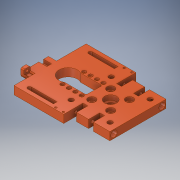
# Autodesk Inventor part: КВ33.044.901 - Щека каретки Z
Saved by Autodesk Inventor 2019 (Build 230136000, 136)
## iProperties
Created: 2019-08-08
Part Number: КВ33.044.901 - Щека каретки Z
Material: Пластик АБС
Document SubType Name: Modeling
Designer: user
Density: 1.06 g/cm^3
Appearance: Гладкий — светло-оранжевый
Mass: 66.5438 g
Surface Area: 300.742 cm^2
Volume: 62.7772 cm^3
Author: user
Autodesk Inventor part; units mm, degrees
(part 1 of 2)
ref_plane "YZ Plane" through (0, 0, 0) normal (1, 0, 0) x (0, 1, 0)
ref_plane "XZ Plane" through (0, 0, 0) normal (0, 1, 0) x (-1, 0, 0)
ref_plane "XY Plane" through (0, 0, 0) normal (0, 0, 1) x (1, 0, 0)
sketch "Эскиз4" plane through (0, 0, 0) normal (0, 1, 0) x (-1, 0, 0)
  circle A0 centre (-24.3, 25) radius 3
  circle A1 centre (24.3, 25) radius 3
  circle A2 centre (24.3, -25) radius 3
  circle A3 centre (-24.3, -25) radius 3
  line L0 (13.5, -21) -> (13.5, -35)
  line L1 (13.5, -35) -> (34, -35)
  line L2 (34, -35) -> (34, 35)
  line L3 (34, 35) -> (13.5, 35)
  line L4 (13.5, 35) -> (13.5, 21)
  line L5 (13.5, 21) -> (7.5, 21)
  line L6 (7.5, 21) -> (7.5, 35)
  line L7 (7.5, 35) -> (-7.5, 35)
  line L8 (-7.5, 35) -> (-7.5, 21)
  line L9 (-7.5, 21) -> (-13.5, 21)
  line L10 (-13.5, 21) -> (-13.5, 35)
  line L11 (-13.5, 35) -> (-34, 35)
  line L12 (-34, 35) -> (-34, -35)
  line L13 (-34, -35) -> (-13.5, -35)
  line L14 (-13.5, -35) -> (-13.5, -21)
  line L15 (-13.5, -21) -> (-7.5, -21)
  line L16 (-7.5, -21) -> (-7.5, -35)
  line L17 (-7.5, -35) -> (7.5, -35)
  line L18 (7.5, -35) -> (7.5, -21)
  line L19 (7.5, -21) -> (13.5, -21)
  circle A4 centre (0, 0) radius 7.5
  circle A5 centre (-11.749999, 11.750148) radius 4.65
  circle A6 centre (-11.750148, -11.749999) radius 4.65
  line L20 (26, 12) -> (16.393422, 12)
  line L21 (26, -12) -> (26, 12)
  line L22 (16.393281, -12) -> (26, -12)
  arc A7 (16, -9.863355) -> (16.393281, -12) centre (11.749999, -11.750148) ccw
  line L23 (16, -9.863355) -> (16, 9.86287)
  arc A8 (16.393422, 12) -> (16, 9.86287) centre (11.750148, 11.749999) ccw
  circle A9 centre (-11.749999, 11.750148) radius 2.6
  circle A10 centre (-11.750148, -11.749999) radius 2.6
  circle A11 centre (11.749999, -11.750148) radius 2.6
  circle A12 centre (11.750148, 11.749999) radius 2.6
  circle A13 centre (0, 0) radius 4.1
  circle A14 centre (11.750148, 11.749999) radius 4.65
  circle A15 centre (11.749999, -11.750148) radius 4.65
  constraints: 48 end point, 14 centre point, 4 point on circle, 2 coincident, 6 other
sketch "Эскиз4 outline for Выдавливание3" plane through (0, 0, 0) normal (0, 1, 0) x (-1, 0, 0)
  line L0 (7.5, -21) -> (13.5, -21)
  line L1 (7.5, -35) -> (7.5, -21)
  line L2 (13.5, -21) -> (13.5, -35)
  line L3 (-7.5, -35) -> (7.5, -35)
  line L4 (13.5, -35) -> (34, -35)
  line L5 (-7.5, -21) -> (-7.5, -35)
  line L6 (34, -35) -> (34, 35)
  line L7 (-13.5, -21) -> (-7.5, -21)
  line L8 (34, 35) -> (13.5, 35)
  line L9 (-13.5, -35) -> (-13.5, -21)
  line L10 (13.5, 35) -> (13.5, 21)
  line L11 (-34, -35) -> (-13.5, -35)
  line L12 (13.5, 21) -> (7.5, 21)
  line L13 (-34, 35) -> (-34, -35)
  line L14 (7.5, 21) -> (7.5, 35)
  line L15 (-13.5, 35) -> (-34, 35)
  line L16 (7.5, 35) -> (-7.5, 35)
  line L17 (-13.5, 21) -> (-13.5, 35)
  line L18 (-7.5, 35) -> (-7.5, 21)
  line L19 (-7.5, 21) -> (-13.5, 21)
  circle A0 centre (-24.3, -25) radius 3
  circle A1 centre (-11.750148, -11.749999) radius 2.6
  circle A2 centre (24.3, -25) radius 3
  circle A3 centre (11.749999, -11.750148) radius 2.6
  circle A4 centre (-11.749999, 11.750148) radius 2.6
  circle A5 centre (-24.3, 25) radius 3
  circle A6 centre (0, 0) radius 4.1
  circle A7 centre (11.750148, 11.749999) radius 2.6
  circle A8 centre (24.3, 25) radius 3
extrude "Выдавливание3" add sketch "Эскиз4 outline for Выдавливание3" along normal blind 10
sketch "Эскиз5" plane through (0, 10, 0) normal (0, 1, 0) x (1, 0, 0)
  circle A0 centre (-24.3, 25) radius 3
  circle A1 centre (24.3, 25) radius 3
  circle A2 centre (24.3, -25) radius 3
  circle A3 centre (-24.3, -25) radius 3
  line L0 (13.5, -21) -> (13.5, -35)
  line L1 (13.5, -35) -> (34, -35)
  line L2 (34, -35) -> (34, 35)
  line L3 (34, 35) -> (13.5, 35)
  line L4 (13.5, 35) -> (13.5, 21)
  line L5 (13.5, 21) -> (7.5, 21)
  line L6 (7.5, 21) -> (7.5, 35)
  line L7 (7.5, 35) -> (-7.5, 35)
  line L8 (-7.5, 35) -> (-7.5, 21)
  line L9 (-7.5, 21) -> (-13.5, 21)
  line L10 (-13.5, 21) -> (-13.5, 35)
  line L11 (-13.5, 35) -> (-34, 35)
  line L12 (-34, 35) -> (-34, -35)
  line L13 (-34, -35) -> (-13.5, -35)
  line L14 (-13.5, -35) -> (-13.5, -21)
  line L15 (-13.5, -21) -> (-7.5, -21)
  line L16 (-7.5, -21) -> (-7.5, -35)
  line L17 (-7.5, -35) -> (7.5, -35)
  line L18 (7.5, -35) -> (7.5, -21)
  line L19 (7.5, -21) -> (13.5, -21)
  circle A4 centre (0, 0) radius 7.5
  circle A5 centre (-11.749999, 11.750148) radius 4.65
  circle A6 centre (-11.750148, -11.749999) radius 4.65
  line L20 (26, 12) -> (16.393422, 12)
  line L21 (26, -12) -> (26, 12)
  line L22 (16.393281, -12) -> (26, -12)
  arc A7 (16, -9.863355) -> (16.393281, -12) centre (11.749999, -11.750148) ccw
  line L23 (16, -9.863355) -> (16, 9.86287)
  arc A8 (16.393422, 12) -> (16, 9.86287) centre (11.750148, 11.749999) ccw
  circle A9 centre (-11.749999, 11.750148) radius 2.6
  circle A10 centre (-11.750148, -11.749999) radius 2.6
  circle A11 centre (11.749999, -11.750148) radius 2.6
  circle A12 centre (11.750148, 11.749999) radius 2.6
  circle A13 centre (0, 0) radius 4.1
  circle A14 centre (11.749999, -11.750148) radius 2.6
  circle A15 centre (11.749999, -11.750148) radius 4.65
  circle A16 centre (11.750148, 11.749999) radius 4.65
  constraints: 48 end point, 16 centre point, 4 point on circle, 2 coincident, 2 concentric
sketch "Эскиз5 outline for Выдавливание4" plane through (0, 10, 0) normal (0, 1, 0) x (1, 0, 0)
  circle A0 centre (-11.749999, 11.750148) radius 4.65
  circle A1 centre (-11.749999, 11.750148) radius 2.6
  circle A2 centre (-11.750148, -11.749999) radius 4.65
  circle A3 centre (-11.750148, -11.749999) radius 2.6
  circle A4 centre (11.749999, -11.750148) radius 4.65
  circle A5 centre (11.749999, -11.750148) radius 2.6
  circle A6 centre (11.750148, 11.749999) radius 4.65
  circle A7 centre (11.750148, 11.749999) radius 2.6
extrude "Выдавливание4" cut sketch "Эскиз5 outline for Выдавливание4" against normal blind 4
sketch "Эскиз6" plane through (0, 10, 0) normal (0, 1, 0) x (1, 0, 0)
  circle A0 centre (-24.3, 25) radius 3
  circle A1 centre (24.3, 25) radius 3
  circle A2 centre (24.3, -25) radius 3
  circle A3 centre (-24.3, -25) radius 3
  line L0 (13.5, -21) -> (13.5, -35)
  line L1 (13.5, -35) -> (34, -35)
  line L2 (34, -35) -> (34, 35)
  line L3 (34, 35) -> (13.5, 35)
  line L4 (13.5, 35) -> (13.5, 21)
  line L5 (13.5, 21) -> (7.5, 21)
  line L6 (7.5, 21) -> (7.5, 35)
  line L7 (7.5, 35) -> (-7.5, 35)
  line L8 (-7.5, 35) -> (-7.5, 21)
  line L9 (-7.5, 21) -> (-13.5, 21)
  line L10 (-13.5, 21) -> (-13.5, 35)
  line L11 (-13.5, 35) -> (-34, 35)
  line L12 (-34, 35) -> (-34, -35)
  line L13 (-34, -35) -> (-13.5, -35)
  line L14 (-13.5, -35) -> (-13.5, -21)
  line L15 (-13.5, -21) -> (-7.5, -21)
  line L16 (-7.5, -21) -> (-7.5, -35)
  line L17 (-7.5, -35) -> (7.5, -35)
  line L18 (7.5, -35) -> (7.5, -21)
  line L19 (7.5, -21) -> (13.5, -21)
  circle A4 centre (0, 0) radius 7.5
  circle A5 centre (-11.749999, 11.750148) radius 4.65
  circle A6 centre (-11.750148, -11.749999) radius 4.65
  line L20 (26, 12) -> (16.393422, 12)
  line L21 (26, -12) -> (26, 12)
  line L22 (16.393281, -12) -> (26, -12)
  arc A7 (16, -9.863355) -> (16.393281, -12) centre (11.749999, -11.750148) ccw
  line L23 (16, -9.863355) -> (16, 9.86287)
  arc A8 (16.393422, 12) -> (16, 9.86287) centre (11.750148, 11.749999) ccw
  circle A9 centre (-11.749999, 11.750148) radius 2.6
  circle A10 centre (-11.750148, -11.749999) radius 2.6
  circle A11 centre (11.749999, -11.750148) radius 2.6
  circle A12 centre (11.750148, 11.749999) radius 2.6
  circle A13 centre (0, 0) radius 4.1
  constraints: 48 end point, 14 centre point, 4 point on circle
sketch "Эскиз6 outline for Выдавливание5" plane through (0, 10, 0) normal (0, 1, 0) x (1, 0, 0)
  circle A0 centre (0, 0) radius 7.5
  circle A1 centre (0, 0) radius 4.1
extrude "Выдавливание5" cut sketch "Эскиз6 outline for Выдавливание5" against normal blind 6
sketch "Эскиз7" plane through (34, 0, 35) normal (1, 0, 0) x (0, 0, -1)
  circle A0 centre (5, 5) radius 2
  circle A1 centre (5, 5) radius 4
  circle A2 centre (65, 5) radius 4
  circle A3 centre (5, 5) radius 4
  line L0 (0, 0) -> (70, 0)
  line L1 (70, 0) -> (70, 10)
  line L2 (0, 10) -> (70, 10)
  line L3 (0, 0) -> (0, 10)
  circle A4 centre (65, 5) radius 2
  circle A5 centre (65, 5) radius 4
  point P0 (35, 0)
  point P1 (35, 0)
  constraints: 8 end point, 6 centre point
sketch "Эскиз7 outline for Выдавливание6" plane through (34, 0, 35) normal (1, 0, 0) x (0, 0, -1)
  circle A0 centre (5, 5) radius 2
  circle A1 centre (65, 5) radius 2
extrude "Выдавливание6" cut sketch "Эскиз7 outline for Выдавливание6" against normal blind 269
sketch "Эскиз8" plane through (34, 0, 35) normal (1, 0, 0) x (0, 0, -1)
  circle A0 centre (5, 5) radius 2
  circle A1 centre (5, 5) radius 4
  circle A2 centre (65, 5) radius 4
  circle A3 centre (5, 5) radius 4
  line L0 (0, 0) -> (70, 0)
  line L1 (70, 0) -> (70, 10)
  line L2 (0, 10) -> (70, 10)
  line L3 (0, 0) -> (0, 10)
  circle A4 centre (65, 5) radius 2
  circle A5 centre (65, 5) radius 4
  point P0 (35, 0)
  point P1 (35, 0)
  constraints: 8 end point, 6 centre point
sketch "Эскиз8 outline for Выдавливание7" plane through (34, 0, 35) normal (1, 0, 0) x (0, 0, -1)
  circle A0 centre (5, 5) radius 4
  circle A1 centre (5, 5) radius 2
  circle A2 centre (65, 5) radius 4
  circle A3 centre (65, 5) radius 2
extrude "Выдавливание7" cut sketch "Эскиз8 outline for Выдавливание7" against normal blind 15
sketch "Эскиз9" plane through (-34, 0, -35) normal (-1, 0, 0) x (0, 0, 1)
  circle A0 centre (5, 5) radius 2
  circle A1 centre (5, 5) radius 4
  circle A2 centre (65, 5) radius 4
  circle A3 centre (5, 5) radius 4
  line L0 (0, 0) -> (70, 0)
  line L1 (70, 0) -> (70, 10)
  line L2 (0, 10) -> (70, 10)
  line L3 (0, 0) -> (0, 10)
  circle A4 centre (65, 5) radius 2
  circle A5 centre (65, 5) radius 4
  point P0 (35, 0)
  point P1 (35, 0)
  constraints: 8 end point, 6 centre point
sketch "Эскиз9 outline for Выдавливание8" plane through (-34, 0, -35) normal (-1, 0, 0) x (0, 0, 1)
  circle A0 centre (5, 5) radius 4
  circle A1 centre (5, 5) radius 2
  circle A2 centre (65, 5) radius 4
  circle A3 centre (65, 5) radius 2
extrude "Выдавливание8" cut sketch "Эскиз9 outline for Выдавливание8" against normal blind 15
sketch "Эскиз17" plane through (-34, 0, -35) normal (-1, 0, 0) x (0, 0, 1)
  line L0 (14, 10) -> (0, 10) projected
  line L1 (70, 0) -> (56, 0) projected
  line L2 (0, 10) -> (70, 10)
  line L3 (70, 10) -> (70, 0)
  line L4 (70, 0) -> (0, 0)
  line L5 (0, 0) -> (0, 10)
  point P0 (35, 0)
  constraints: 8 end point, 2 parallel, 1 horizontal, 1 perpendicular
sketch "Эскиз17 outline for Выдавливание14" plane through (-34, 0, -35) normal (-1, 0, 0) x (0, 0, 1)
  line L0 (0, 10) -> (70, 10)
  line L1 (70, 10) -> (70, 0)
  line L2 (70, 0) -> (0, 0)
  line L3 (0, 0) -> (0, 10)
extrude "Выдавливание14" add sketch "Эскиз17 outline for Выдавливание14" along normal blind 33
sketch "Эскиз18" plane through (0, 0, 0) normal (0, -1, 0) x (1, 0, 0)
  line L0 (-35.2, -12.6) -> (-35.2, -14.9)
  line L1 (-35.2, -12.6) -> (-33.8, -12.6)
  line L2 (-33.8, -14.9) -> (-33.8, -12.6)
  line L3 (-27.2, -14.9) -> (-33.8, -14.9)
  line L4 (-27.2, -12.6) -> (-27.2, -14.9)
  circle A0 centre (-53, 0) radius 9.15
  circle A1 centre (-53, 0) radius 1.5
  circle A2 centre (-17, 8) radius 1.3
  circle A3 centre (-30.5, 13.5) radius 1.3
  circle A4 centre (-22.5, 13.5) radius 1.3
  circle A5 centre (-38.5, 13.5) radius 1.3
  circle A6 centre (-46.5, 13.5) radius 1.3
  circle A7 centre (-17, -8) radius 1.3
  circle A8 centre (-30.5, -13.5) radius 1.3
  circle A9 centre (-22.5, -13.5) radius 1.3
  circle A10 centre (-38.5, -13.5) radius 1.3
  circle A11 centre (-46.5, -13.5) radius 1.3
  line L5 (-64.019804, -0.1) -> (-63.479583, -0.1)
  line L6 (-64.019804, -7) -> (-64.019804, -0.1)
  arc A12 (-64.019804, -7) -> (-63.968614, -7.75) centre (-58.5, -7) ccw
  line L7 (-61.5, -7.75) -> (-63.968614, -7.75)
  arc A13 (-59.75, -9.5) -> (-61.5, -7.75) centre (-61.5, -9.5) ccw
  line L8 (-59.75, -10) -> (-59.75, -9.5)
  line L9 (-22.193741, -10) -> (-59.75, -10)
  arc A14 (-22.193741, -10) -> (-21.505509, -9.607843) centre (-22.193741, -9.2) ccw
  arc A15 (-21.505509, -9.607843) -> (-20.892157, -8.994491) centre (-20, -10.5) ccw
  arc A16 (-20.892157, -8.994491) -> (-20.5, -8.306259) centre (-21.3, -8.306259) ccw
  line L10 (-20.5, 8.306259) -> (-20.5, -8.306259)
  arc A17 (-20.5, 8.306259) -> (-20.892157, 8.994491) centre (-21.3, 8.306259) ccw
  arc A18 (-21.505509, 9.607843) -> (-20.892157, 8.994491) centre (-20, 10.5) ccw
  arc A19 (-20.892157, 8.994491) -> (-21.505509, 9.607843) centre (-20, 10.5) ccw
  line L11 (-59.75, -11.322904) -> (-59.75, -10)
  arc A20 (-59.75, -11.322904) -> (-58.5, -11.5) centre (-58.498893, -6.992184) ccw
  line L12 (-58.5, -11.5) -> (-51, -11.5)
  line L13 (-51, -12.6) -> (-51, -11.5)
  line L14 (-49.8, -12.6) -> (-51, -12.6)
  line L15 (-49.8, -14.9) -> (-49.8, -12.6)
  line L16 (-43.2, -14.9) -> (-49.8, -14.9)
  line L17 (-43.2, -12.6) -> (-43.2, -14.9)
  line L18 (-41.8, -12.6) -> (-43.2, -12.6)
  line L19 (-41.8, -14.9) -> (-41.8, -12.6)
  line L20 (-35.2, -14.9) -> (-41.8, -14.9)
  line L21 (-35.2, -12.6) -> (-35.2, -14.9)
  line L22 (-33.8, -12.6) -> (-35.2, -12.6)
  line L23 (-33.8, -14.9) -> (-33.8, -12.6)
  line L24 (-27.2, -14.9) -> (-33.8, -14.9)
  line L25 (-27.2, -12.6) -> (-27.2, -14.9)
  line L26 (-25.8, -12.6) -> (-27.2, -12.6)
  line L27 (-25.8, -14.9) -> (-25.8, -12.6)
  line L28 (-19.2, -14.9) -> (-25.8, -14.9)
  line L29 (-19.2, -12.6) -> (-19.2, -14.9)
  line L30 (-17.980196, -12.6) -> (-19.2, -12.6)
  arc A21 (-17.980196, -12.6) -> (-17.899999, -12.519803) centre (-19, -11.5) ccw
  line L31 (-17.899999, -11.3) -> (-17.899999, -12.519803)
  line L32 (-15.6, -11.3) -> (-17.899999, -11.3)
  line L33 (-15.6, -4.7) -> (-15.6, -11.3)
  line L34 (-17.9, -4.7) -> (-15.6, -4.7)
  line L35 (-17.9, 4.7) -> (-17.9, -4.7)
  line L36 (-15.6, 4.7) -> (-17.9, 4.7)
  line L37 (-15.6, 11.3) -> (-15.6, 4.7)
  line L38 (-17.9, 11.3) -> (-15.6, 11.3)
  line L39 (-17.9, 12.519804) -> (-17.9, 11.3)
  arc A22 (-17.9, 12.519804) -> (-17.980197, 12.600001) centre (-19, 11.5) ccw
  line L40 (-19.2, 12.600001) -> (-17.980197, 12.600001)
  line L41 (-19.2, 14.9) -> (-19.2, 12.600001)
  line L42 (-25.8, 14.9) -> (-19.2, 14.9)
  line L43 (-25.8, 12.6) -> (-25.8, 14.9)
  line L44 (-27.2, 12.6) -> (-25.8, 12.6)
  line L45 (-27.2, 14.9) -> (-27.2, 12.6)
  line L46 (-33.8, 14.9) -> (-27.2, 14.9)
  line L47 (-33.8, 12.6) -> (-33.8, 14.9)
  line L48 (-35.2, 12.6) -> (-33.8, 12.6)
  line L49 (-35.2, 14.9) -> (-35.2, 12.6)
  line L50 (-41.8, 14.9) -> (-35.2, 14.9)
  line L51 (-41.8, 12.6) -> (-41.8, 14.9)
  line L52 (-43.2, 12.6) -> (-41.8, 12.6)
  line L53 (-43.2, 14.9) -> (-43.2, 12.6)
  line L54 (-49.8, 14.9) -> (-43.2, 14.9)
  line L55 (-49.8, 12.6) -> (-49.8, 14.9)
  line L56 (-51, 12.6) -> (-49.8, 12.6)
  line L57 (-51, 11.5) -> (-51, 12.6)
  line L58 (-58.5, 11.5) -> (-51, 11.5)
  arc A23 (-58.5, 11.5) -> (-59.75, 11.322904) centre (-58.498893, 6.992184) ccw
  line L59 (-59.75, 10) -> (-59.75, 11.322904)
  line L60 (-59.75, 9.5) -> (-59.75, 10)
  arc A24 (-61.5, 7.75) -> (-59.75, 9.5) centre (-61.5, 9.5) ccw
  line L61 (-63.968614, 7.75) -> (-61.5, 7.75)
  arc A25 (-63.968614, 7.75) -> (-64.019804, 7) centre (-58.5, 7) ccw
  line L62 (-64.019804, 0.1) -> (-64.019804, 7)
  line L63 (-63.479583, 0.1) -> (-64.019804, 0.1)
  arc A26 (-20.892157, -8.994491) -> (-21.505509, -9.607843) centre (-20, -10.5) ccw
  arc A27 (-21.505509, 9.607843) -> (-22.193741, 10) centre (-22.193741, 9.2) ccw
  line L64 (-59.75, 10) -> (-22.193741, 10)
  line L65 (0, 0) -> (-34, 0)
  line L66 (-34, 0) -> (-53, 0)
  line L67 (-53, -9.15) -> (-53, -10)
  line L68 (-53, 10) -> (-53, 9.15)
  dimension "d62" = 34
  dimension "d63" = 19
  constraints: 138 end point, 34 point on circle, 28 centre point, 4 point on line, 2 horizontal, 1 perpendicular
  measures "d62" distance of L65.start L65.end
  measures "d63" distance of L65.end L66.end
sketch "Эскиз18 outline for Выдавливание15" plane through (0, 0, 0) normal (0, -1, 0) x (1, 0, 0)
  arc A0 (-53, 9.15) -> (-53, -9.15) centre (-53, 0) ccw
  line L0 (-53, -9.15) -> (-53, -10)
  line L1 (-53, -10) -> (-22.193741, -10)
  arc A1 (-22.193741, -10) -> (-21.505509, -9.607843) centre (-22.193741, -9.2) ccw
  arc A2 (-21.505509, -9.607843) -> (-20.892157, -8.994491) centre (-20, -10.5) cw
  arc A3 (-20.892157, -8.994491) -> (-20.5, -8.306259) centre (-21.3, -8.306259) ccw
  line L2 (-20.5, -8.306259) -> (-20.5, 8.306259)
  arc A4 (-20.5, 8.306259) -> (-20.892157, 8.994491) centre (-21.3, 8.306259) ccw
  arc A5 (-20.892157, 8.994491) -> (-21.505509, 9.607843) centre (-20, 10.5) cw
  arc A6 (-21.505509, 9.607843) -> (-22.193741, 10) centre (-22.193741, 9.2) ccw
  line L3 (-22.193741, 10) -> (-53, 10)
  line L4 (-53, 10) -> (-53, 9.15)
  circle A7 centre (-30.5, 13.5) radius 1.3
  circle A8 centre (-22.5, 13.5) radius 1.3
  circle A9 centre (-38.5, 13.5) radius 1.3
  circle A10 centre (-46.5, 13.5) radius 1.3
  circle A11 centre (-30.5, -13.5) radius 1.3
  circle A12 centre (-22.5, -13.5) radius 1.3
  circle A13 centre (-38.5, -13.5) radius 1.3
  circle A14 centre (-46.5, -13.5) radius 1.3
extrude "Выдавливание15" cut sketch "Эскиз18 outline for Выдавливание15" against normal blind 23
sketch "Эскиз19" plane through (0, 0, 0) normal (0, -1, 0) x (1, 0, 0)
  arc A0 (-53, 9.15) -> (-53, -9.15) centre (-53, 0) ccw projected
  circle A1 centre (-53, 0) radius 11.5
  point P0 (0, 0)
  dimension "d66" = 23
  constraints: 1 centre point, 1 coincident
  measures "d66" diameter of A1
sketch "Эскиз19 outline for Выдавливание16" plane through (0, 0, 0) normal (0, -1, 0) x (1, 0, 0)
  circle A0 centre (-53, 0) radius 11.5
extrude "Выдавливание16" cut sketch "Эскиз19 outline for Выдавливание16" against normal blind 23
sketch "Эскиз20" plane through (0, 10, 0) normal (0, 1, 0) x (1, 0, 0)
  circle A0 centre (-22.5, -13.5) radius 1.3 projected
  circle A1 centre (-22.5, -13.5) radius 2.5
  circle A2 centre (-30.5, -13.5) radius 1.3 projected
  circle A3 centre (-30.5, -13.5) radius 2.5
  circle A4 centre (-38.5, -13.5) radius 1.3 projected
  circle A5 centre (-38.5, -13.5) radius 2.5
  circle A6 centre (-46.5, -13.5) radius 1.3 projected
  circle A7 centre (-46.5, -13.5) radius 2.5
  circle A8 centre (-46.5, 13.5) radius 1.3 projected
  circle A9 centre (-46.5, 13.5) radius 2.5
  circle A10 centre (-38.5, 13.5) radius 1.3 projected
  circle A11 centre (-38.5, 13.5) radius 2.5
  circle A12 centre (-30.5, 13.5) radius 1.3 projected
  circle A13 centre (-30.5, 13.5) radius 2.5
  circle A14 centre (-22.5, 13.5) radius 1.3 projected
  circle A15 centre (-22.5, 13.5) radius 2.5
  point P0 (0, 0)
  dimension "d69" = 5
  dimension "d70" = 5
  dimension "d71" = 5
  dimension "d72" = 5
  dimension "d73" = 5
  dimension "d74" = 5
  dimension "d75" = 5
  dimension "d76" = 5
  constraints: 8 centre point, 8 coincident
  measures "d69" diameter of A1
  measures "d70" diameter of A3
  measures "d71" diameter of A5
  measures "d72" diameter of A7
  measures "d73" diameter of A9
  measures "d74" diameter of A11
  measures "d75" diameter of A13
  measures "d76" diameter of A15
sketch "Эскиз20 outline for Выдавливание17" plane through (0, 10, 0) normal (0, 1, 0) x (1, 0, 0)
  circle A0 centre (-22.5, -13.5) radius 2.5
  circle A1 centre (-30.5, -13.5) radius 2.5
  circle A2 centre (-38.5, -13.5) radius 2.5
  circle A3 centre (-46.5, -13.5) radius 2.5
  circle A4 centre (-46.5, 13.5) radius 2.5
  circle A5 centre (-38.5, 13.5) radius 2.5
  circle A6 centre (-30.5, 13.5) radius 2.5
  circle A7 centre (-22.5, 13.5) radius 1.3
extrude "Выдавливание17" cut sketch "Эскиз20 outline for Выдавливание17" against normal blind 2
move faces "Перенос3" translate (0, 0, -10) faces at (-49.166667, 6.666667, -35)
move faces "Перенос4" translate (0, 0, 10) faces at (-31.333333, 6.666667, 35)
sketch "Эскиз21" plane through (0, 10, 0) normal (0, 1, 0) x (1, 0, 0)
  line L0 (-13.5, -45) -> (-67, -45)
  line L1 (-40.25, -45) -> (-40.25, -38)
  line L2 (-13.5, 45) -> (-67, 45)
  line L3 (-40.25, 45) -> (-40.25, 38)
  line L4 (-17.168403, -38) -> (-63.331597, -38) construction
  line L5 (-17.168403, -35.75) -> (-63.331597, -35.75)
  line L6 (-63.331597, -40.25) -> (-17.168403, -40.25)
  arc A0 (-17.168403, -40.25) -> (-17.168403, -35.75) centre (-17.168403, -38) ccw
  arc A1 (-63.331597, -35.75) -> (-63.331597, -40.25) centre (-63.331597, -38) ccw
  line L7 (-17.168403, 38) -> (-63.331597, 38) construction
  line L8 (-17.168403, 40.25) -> (-63.331597, 40.25)
  line L9 (-63.331597, 35.75) -> (-17.168403, 35.75)
  arc A2 (-17.168403, 35.75) -> (-17.168403, 40.25) centre (-17.168403, 38) ccw
  arc A3 (-63.331597, 40.25) -> (-63.331597, 35.75) centre (-63.331597, 38) ccw
  point P0 (0, 0)
  dimension "d85" = 7
  dimension "d86" = 7
  dimension "d87" = 90
  dimension "d88" = 4.5
  dimension "d89" = 4.5
  constraints: 20 end point, 8 point on circle, 8 tangent, 4 centre point, 4 midpoint, 2 horizontal, 2 parallel, 1 vertical
  measures "d85" distance of L1.start L1.end
  measures "d86" distance of L3.start L3.end
  measures "d87" angle of L2 L3
  measures "d88" diameter of A1
  measures "d89" diameter of A3
sketch "Эскиз21 outline for Выдавливание18" plane through (0, 10, 0) normal (0, 1, 0) x (1, 0, 0)
  arc A0 (-17.168403, -40.25) -> (-17.168403, -35.75) centre (-17.168403, -38) ccw
  line L0 (-63.331597, -40.25) -> (-17.168403, -40.25)
  arc A1 (-63.331597, -35.75) -> (-63.331597, -40.25) centre (-63.331597, -38) ccw
  line L1 (-17.168403, -35.75) -> (-63.331597, -35.75)
  arc A2 (-17.168403, 35.75) -> (-17.168403, 40.25) centre (-17.168403, 38) ccw
  line L2 (-63.331597, 35.75) -> (-17.168403, 35.75)
  arc A3 (-63.331597, 40.25) -> (-63.331597, 35.75) centre (-63.331597, 38) ccw
  line L3 (-17.168403, 40.25) -> (-63.331597, 40.25)
extrude "Выдавливание18" cut sketch "Эскиз21 outline for Выдавливание18" against normal blind 15.5
move faces "Перенос5" translate (-8.5, 0, 0) faces at (-67, 3.333333, 15)
sketch "Эскиз24" plane through (-75.5, 0, -45) normal (-1, 0, 0) x (0, 0, 1)
  line L0 (90, 0) -> (90, 10) projected
  line L1 (90, 0) -> (66, 0) projected
  line L2 (90, 0) -> (90, 5.8)
  line L3 (90, 5.8) -> (49.1, 5.8)
  line L4 (49.1, 5.8) -> (90, 5.8)
  line L5 (90, 5.8) -> (90, 10)
  line L6 (90, 10) -> (49.1, 10)
  line L7 (49.1, 10) -> (49.1, 5.8)
  line L8 (49.1, 10) -> (71.6, 10)
  line L9 (90, 10) -> (0, 10) projected
  line L10 (71.6, 10) -> (71.6, 5.8)
  point P0 (45, 0)
  dimension "d103" = 5.8
  dimension "d104" = 40.9
  dimension "d105" = 22.5
  constraints: 16 end point, 3 perpendicular, 3 point on line, 2 parallel, 1 horizontal
  measures "d103" distance of L0.start L2.end
  measures "d104" distance of L2.end L3.end
  measures "d105" distance of L6.end L8.end
sketch "Эскиз24 outline for Выдавливание20" plane through (-75.5, 0, -45) normal (-1, 0, 0) x (0, 0, 1)
  line L0 (49.1, 10) -> (49.1, 5.8)
  line L1 (71.6, 10) -> (49.1, 10)
  line L2 (71.6, 5.8) -> (71.6, 10)
  line L3 (49.1, 5.8) -> (71.6, 5.8)
extrude "Выдавливание20" add sketch "Эскиз24 outline for Выдавливание20" along normal blind 10
sketch "Эскиз25" plane through (-75.5, 0, -45) normal (-1, 0, 0) x (0, 0, 1)
  line L0 (49.1, 5.8) -> (49.1, 10)
  line L1 (49.1, 5.8) -> (43.1, 5.8)
  line L2 (43.1, 5.8) -> (43.1, 0)
  line L3 (43.1, 0) -> (49.1, 0)
  line L4 (49.1, 0) -> (49.1, 5.8)
  line L5 (43.1, 5.8) -> (37.1, 5.8)
  line L6 (37.1, 5.8) -> (37.1, 10)
  line L7 (37.1, 10) -> (43.1, 10)
  line L8 (43.1, 10) -> (43.1, 5.8)
  line L9 (41.995544, 5.8) -> (43.1, 4.63325)
  line L10 (49.1, 4.63325) -> (50.332559, 5.8)
  line L11 (71.6, 5.8) -> (49.1, 5.8)
  line L12 (49.1, 5.8) -> (50.332559, 5.8)
  point P0 (45, 0)
  dimension "d108" = 6
  dimension "d109" = 5.8
  dimension "d110" = 6
  dimension "d111" = 4.2
  constraints: 22 end point, 4 parallel, 4 point on line, 3 horizontal, 3 perpendicular
  measures "d108" distance of L3.end L2.end
  measures "d109" distance of L2.end L1.end
  measures "d110" distance of L6.end L7.end
  measures "d111" distance of L5.end L6.end
sketch "Эскиз25 outline for Выдавливание21" plane through (-75.5, 0, -45) normal (-1, 0, 0) x (0, 0, 1)
  line L0 (41.995544, 5.8) -> (43.1, 4.63325)
  line L1 (43.1, 4.63325) -> (43.1, 0)
  line L2 (43.1, 0) -> (49.1, 0)
  line L3 (49.1, 0) -> (49.1, 4.63325)
  line L4 (49.1, 4.63325) -> (50.332559, 5.8)
  line L5 (50.332559, 5.8) -> (43.1, 5.8)
  line L6 (43.1, 5.8) -> (43.1, 10)
  line L7 (43.1, 10) -> (37.1, 10)
  line L8 (37.1, 10) -> (37.1, 5.8)
  line L9 (37.1, 5.8) -> (41.995544, 5.8)
extrude "Выдавливание21" add sketch "Эскиз25 outline for Выдавливание21" along normal blind 10
sketch "Эскиз26" plane through (-85.5, 0, -45) normal (-1, 0, 0) x (0, 0, 1)
  line L0 (71.6, 5.8) -> (71.6, 10) projected
  line L1 (71.6, 7.9) -> (67.5, 7.9)
  line L2 (71.6, 5.8) -> (63.6, 5.8)
  line L3 (63.6, 5.8) -> (63.6, 15.1)
  line L4 (63.6, 15.1) -> (71.6, 15.1)
  line L5 (71.6, 15.1) -> (71.6, 5.8)
  line L6 (67.5, 7.9) -> (67.5, 11.7)
  circle A0 centre (67.5, 11.7) radius 1.5
  point P0 (45, 0)
  dimension "d114" = 4.1
  dimension "d115" = 8
  dimension "d116" = 9.3
  dimension "d117" = 3.8
  dimension "d118" = 3
  constraints: 12 end point, 2 horizontal, 2 parallel, 1 centre point, 1 coincident, 1 midpoint, 1 perpendicular, 1 vertical
  measures "d114" distance of L1.start L1.end
  measures "d115" distance of L3.end L4.end
  measures "d116" distance of L2.end L3.end
  measures "d117" distance of L1.end L6.end
  measures "d118" diameter of A0
sketch "Эскиз26 outline for Выдавливание22" plane through (-85.5, 0, -45) normal (-1, 0, 0) x (0, 0, 1)
  line L0 (63.6, 5.8) -> (71.6, 5.8)
  line L1 (63.6, 15.1) -> (63.6, 5.8)
  line L2 (71.6, 5.8) -> (71.6, 15.1)
  line L3 (71.6, 15.1) -> (63.6, 15.1)
  circle A0 centre (67.5, 11.7) radius 1.5
extrude "Выдавливание22" add sketch "Эскиз26 outline for Выдавливание22" against normal blind 4
sketch "Эскиз29" plane through (0, 10, 0) normal (0, 1, 0) x (1, 0, 0)
  line L0 (-81.5, -21) -> (-81.5, -24)
  line L1 (-81.5, -21) -> (-81.5, -20)
  line L2 (-81.5, -18.6) -> (-81.5, -26.6)
  line L3 (-75.5, -26.6) -> (-75.5, -5.332559)
  line L4 (-81.5, -20) -> (-75.5, -20)
  line L5 (-75.5, -20) -> (-75.5, -25)
  line L6 (-75.5, -25) -> (-81.5, -25)
  line L7 (-81.5, -25) -> (-81.5, -20)
  point P0 (0, 0)
  dimension "d127" = 1
  dimension "d128" = 5
  constraints: 10 end point, 2 parallel, 2 point on line, 1 horizontal, 1 perpendicular
  measures "d127" distance of L0.start L1.end
  measures "d128" distance of L4.end L5.end
sketch "Эскиз29 outline for Выдавливание25" plane through (0, 10, 0) normal (0, 1, 0) x (1, 0, 0)
  line L0 (-75.5, -20) -> (-81.5, -20)
  line L1 (-75.5, -25) -> (-75.5, -20)
  line L2 (-81.5, -25) -> (-75.5, -25)
  line L3 (-81.5, -20) -> (-81.5, -25)
extrude "Выдавливание25" cut sketch "Эскиз29 outline for Выдавливание25" against normal blind 2
chamfer "Фаска2" distance 1.25 angle 45 2 edges at (-78.5, 10, 20) (-78.5, 10, 25)
chamfer "Фаска3" distance 1.25 angle 45 2 edges at (-83.5, 15.1, 26.6) (-83.5, 15.1, 18.6)
sketch "Эскиз30" plane through (-75.5, 0, 45) normal (-1, 0, 0) x (0, 0, 1)
  circle A0 centre (-15, 5) radius 2 projected
  circle A1 centre (-15, 5) radius 4
  circle A2 centre (-75, 5) radius 2 projected
  circle A3 centre (-75, 5) radius 4
  point P0 (-45, 0)
  constraints: 2 centre point, 2 coincident
sketch "Эскиз30 outline for Выдавливание26" plane through (-75.5, 0, 45) normal (-1, 0, 0) x (0, 0, 1)
  circle A0 centre (-15, 5) radius 4
  circle A1 centre (-75, 5) radius 4
extrude "Выдавливание26" cut sketch "Эскиз30 outline for Выдавливание26" against normal blind 56.25 and the other way blind 12.125
sketch "Эскиз32" plane through (0, 0, 0) normal (0, -1, 0) x (1, 0, 0)
  line L0 (-13.5, -21) -> (-13.5, -45)
  line L1 (-13.5, -45) -> (-31.053592, -45)
  line L2 (-31.053592, -45) -> (-31.053592, -35.241695)
  line L3 (-31.053592, -35.241695) -> (-13.5, -35.241695)
  line L4 (-13.5, -35.241695) -> (-13.5, -45)
  line L5 (-13.5, 45) -> (-31.053592, 45)
  line L6 (-31.053592, 45) -> (-31.053592, 35)
  line L7 (-31.053592, 35) -> (-13.5, 35)
  line L8 (-13.5, 35) -> (-13.5, 45)
  point P0 (0, 0)
  dimension "d145" = 10
  constraints: 16 end point, 4 parallel, 2 horizontal, 2 perpendicular, 1 point on line
  measures "d145" distance of L7.end L5.start
sketch "Эскиз32 outline for Выдавливание27" plane through (0, 0, 0) normal (0, -1, 0) x (1, 0, 0)
  line L0 (-13.5, -45) -> (-31.053592, -45)
  line L1 (-31.053592, -45) -> (-31.053592, -35.241695)
  line L2 (-31.053592, -35.241695) -> (-13.5, -35.241695)
  line L3 (-13.5, -35.241695) -> (-13.5, -45)
  line L4 (-13.5, 35) -> (-13.5, 45)
  line L5 (-31.053592, 35) -> (-13.5, 35)
  line L6 (-31.053592, 45) -> (-31.053592, 35)
  line L7 (-13.5, 45) -> (-31.053592, 45)
extrude "Выдавливание27" add sketch "Эскиз32 outline for Выдавливание27" against normal blind 10
sketch "Эскиз31" plane through (0, 0, 0) normal (0, -1, 0) x (1, 0, 0)
  line L0 (-11.162974, 50.524965) -> (-11.675559, 50.524965)
  line L1 (-11.675559, 50.524965) -> (-11.767254, 49.090957)
  arc A0 (-15.958694, 49.090957) -> (-11.767254, 49.090957) centre (-13.862974, 49.224965) ccw
  line L2 (-15.958694, 49.090957) -> (-16.05039, 50.524965)
  line L3 (-16.05039, 50.524965) -> (-20.33871, 50.524965)
  arc A1 (-20.33871, 50.524965) -> (-20.409421, 50.495675) centre (-20.33871, 50.424965) ccw
  line L4 (-20.409421, 50.495675) -> (-20.733685, 50.171411)
  arc A2 (-21.087238, 50.024965) -> (-20.733685, 50.171411) centre (-21.087238, 50.524965) ccw
  line L5 (-21.087238, 50.024965) -> (-30.762974, 50.024965)
  arc A3 (-30.762974, 50.024965) -> (-30.862974, 49.924965) centre (-30.762974, 49.924965) ccw
  line L6 (-30.862974, 49.924965) -> (-30.862974, 40.774965)
  arc A4 (-30.862974, 40.774965) -> (-30.762974, 40.674965) centre (-30.762974, 40.774965) ccw
  line L7 (-30.762974, 40.674965) -> (-27.837238, 40.674965)
  arc A5 (-27.483685, 40.528518) -> (-27.837238, 40.674965) centre (-27.837238, 40.174965) ccw
  line L8 (-27.483685, 40.528518) -> (-27.159421, 40.204254)
  arc A6 (-27.159421, 40.204254) -> (-27.08871, 40.174965) centre (-27.08871, 40.274965) ccw
  line L9 (-27.08871, 40.174965) -> (-24.337238, 40.174965)
  arc A7 (-24.337238, 40.174965) -> (-24.266528, 40.204254) centre (-24.337238, 40.274965) ccw
  line L10 (-24.266528, 40.204254) -> (-23.942264, 40.528518)
  arc A8 (-23.58871, 40.674965) -> (-23.942264, 40.528518) centre (-23.58871, 40.174965) ccw
  line L11 (-23.58871, 40.674965) -> (-18.337238, 40.674965)
  arc A9 (-17.983685, 40.528518) -> (-18.337238, 40.674965) centre (-18.337238, 40.174965) ccw
  line L12 (-17.983685, 40.528518) -> (-17.659421, 40.204254)
  arc A10 (-17.659421, 40.204254) -> (-17.58871, 40.174965) centre (-17.58871, 40.274965) ccw
  line L13 (-17.58871, 40.174965) -> (-14.837238, 40.174965)
  arc A11 (-14.837238, 40.174965) -> (-14.766528, 40.204254) centre (-14.837238, 40.274965) ccw
  line L14 (-14.766528, 40.204254) -> (-14.442264, 40.528518)
  arc A12 (-14.08871, 40.674965) -> (-14.442264, 40.528518) centre (-14.08871, 40.174965) ccw
  line L15 (-14.08871, 40.674965) -> (-11.162974, 40.674965)
  arc A13 (-11.162974, 40.674965) -> (-11.062974, 40.774965) centre (-11.162974, 40.774965) ccw
  line L16 (-11.062974, 40.774965) -> (-11.062974, 50.424965)
  arc A14 (-11.062974, 50.424965) -> (-11.162974, 50.524965) centre (-11.162974, 50.424965) ccw
  circle A15 centre (-16.212974, 42.724965) radius 1.25
  circle A16 centre (-25.712974, 42.724965) radius 1.25
  line L17 (-26.886308, 44.974965) -> (-26.269641, 46.274965)
  line L18 (-26.269641, 46.274965) -> (-26.252974, 46.274965)
  line L19 (-26.252974, 46.274965) -> (-25.652974, 44.974965)
  line L20 (-25.652974, 44.974965) -> (-25.779797, 44.974965)
  line L21 (-25.779797, 44.974965) -> (-25.971985, 45.391631)
  line L22 (-25.971985, 45.391631) -> (-26.561308, 45.391631)
  line L23 (-26.561308, 45.391631) -> (-26.758964, 44.974965)
  line L24 (-26.758964, 44.974965) -> (-26.886308, 44.974965)
  spline S0 degree 3 poles (-24.066308, 45.911423) (-24.066544, 45.920293) (-24.067009, 45.937775) (-24.071116, 45.963406) (-24.077323, 45.98813) (-24.086217, 46.012023) (-24.097957, 46.034846) (-24.112247, 46.056625) (-24.128734, 46.077681) (-24.147808, 46.097424) (-24.168761, 46.115506) (-24.190896, 46.131523) (-24.214314, 46.144909) (-24.238918, 46.155882) (-24.264637, 46.16449) (-24.291523, 46.170455) (-24.319501, 46.1742) (-24.338605, 46.174707) (-24.348339, 46.174965) knots 0 0 0 0 0.0619654 0.12212191 0.1809885 0.23993322 0.29990583 0.35998885 0.42177574 0.48657583 0.5515348 0.61501754 0.67725862 0.73972996 0.8030501 0.86649513 0.93197347 1 1 1 1
  spline S1 degree 3 poles (-24.348339, 46.174965) (-24.358505, 46.174699) (-24.37847, 46.174178) (-24.407783, 46.170529) (-24.435746, 46.164235) (-24.46243, 46.155627) (-24.48788, 46.144685) (-24.511973, 46.131056) (-24.534653, 46.114794) (-24.555965, 46.096356) (-24.5756, 46.075828) (-24.592851, 46.052944) (-24.607926, 46.028123) (-24.621078, 46.00143) (-24.631758, 45.972625) (-24.63992, 45.941808) (-24.646378, 45.909114) (-24.648535, 45.886537) (-24.649641, 45.874965) knots 0 0 0 0 0.06443867 0.12654691 0.18688715 0.24587754 0.30404088 0.36219122 0.42097593 0.48066028 0.54060027 0.6006891 0.66193579 0.72444251 0.78903839 0.85631376 0.92635203 1 1 1 1
  line L25 (-24.649641, 45.874965) -> (-24.766308, 45.874965)
  spline S2 degree 3 poles (-24.766308, 45.874965) (-24.765547, 45.890443) (-24.764054, 45.92084) (-24.757061, 45.965161) (-24.747054, 46.007524) (-24.732906, 46.04759) (-24.715335, 46.085713) (-24.694264, 46.121741) (-24.669306, 46.155538) (-24.641001, 46.18679) (-24.610258, 46.215459) (-24.577087, 46.240217) (-24.54223, 46.261135) (-24.505793, 46.278622) (-24.467365, 46.291749) (-24.427294, 46.301488) (-24.385405, 46.307348) (-24.356865, 46.307978) (-24.342349, 46.308298) knots 0 0 0 0 0.06879079 0.13510329 0.19897867 0.2619043 0.32349497 0.38519538 0.44696924 0.50976478 0.57225057 0.63340518 0.69325116 0.75258316 0.81257927 0.87327508 0.93554994 1 1 1 1
  spline S3 degree 3 poles (-24.342349, 46.308298) (-24.328095, 46.307964) (-24.300085, 46.307309) (-24.259204, 46.301677) (-24.220287, 46.292858) (-24.183409, 46.280483) (-24.148864, 46.263849) (-24.116392, 46.243867) (-24.085608, 46.220757) (-24.057897, 46.193548) (-24.032451, 46.164502) (-24.010499, 46.133492) (-23.9917, 46.101464) (-23.97603, 46.068173) (-23.964495, 46.033307) (-23.955737, 45.997372) (-23.950787, 45.959998) (-23.950027, 45.934701) (-23.949641, 45.92184) knots 0 0 0 0 0.06947546 0.1365168 0.20078882 0.26382967 0.32573502 0.38729069 0.44950922 0.51296782 0.57627522 0.6375801 0.69790261 0.75717209 0.81659853 0.87665317 0.93728964 1 1 1 1
  spline S4 degree 3 poles (-23.949641, 45.92184) (-23.95027, 45.903733) (-23.951517, 45.867838) (-23.962182, 45.81509) (-23.978839, 45.763984) (-23.998895, 45.722853) (-24.019128, 45.689709) (-24.037361, 45.662421) (-24.058705, 45.633039) (-24.083471, 45.601661) (-24.111147, 45.568043) (-24.141984, 45.532204) (-24.176201, 45.494514) (-24.200217, 45.468772) (-24.212662, 45.455434) knots 0 0 0 0 0.0987022 0.19567231 0.29242243 0.39134254 0.44446244 0.50422878 0.57035234 0.64254575 0.72228751 0.80792112 0.90046954 1 1 1 1
  line L26 (-24.212662, 45.455434) -> (-24.537922, 45.108298)
  line L27 (-24.537922, 45.108298) -> (-23.932974, 45.108298)
  line L28 (-23.932974, 45.108298) -> (-23.932974, 44.974965)
  line L29 (-23.932974, 44.974965) -> (-24.816308, 44.974965)
  line L30 (-24.816308, 44.974965) -> (-24.312141, 45.512986)
  spline S5 degree 3 poles (-24.312141, 45.512986) (-24.299866, 45.525799) (-24.276288, 45.550412) (-24.242941, 45.586345) (-24.212989, 45.61968) (-24.18624, 45.650355) (-24.163273, 45.678818) (-24.142892, 45.704148) (-24.126562, 45.727457) (-24.108839, 45.754475) (-24.091674, 45.787462) (-24.076923, 45.827775) (-24.067929, 45.869273) (-24.06685, 45.897317) (-24.066308, 45.911423) knots 0 0 0 0 0.11080264 0.2128292 0.30610131 0.39064732 0.46692447 0.53448104 0.59358694 0.644557 0.73620045 0.82502403 0.91198558 1 1 1 1
  line L31 (-23.556308, 45.624965) -> (-23.422974, 46.274965)
  line L32 (-23.422974, 46.274965) -> (-22.889641, 46.274965)
  line L33 (-22.889641, 46.274965) -> (-22.889641, 46.141631)
  line L34 (-22.889641, 46.141631) -> (-23.331828, 46.141631)
  line L35 (-23.331828, 46.141631) -> (-23.401881, 45.799704)
  spline S6 degree 3 poles (-23.401881, 45.799704) (-23.388117, 45.803504) (-23.361452, 45.810866) (-23.322096, 45.819039) (-23.284733, 45.823966) (-23.260488, 45.824639) (-23.248756, 45.824965) knots 0 0 0 0 0.27506837 0.53290146 0.77397346 1 1 1 1
  spline S7 degree 3 poles (-23.248756, 45.824965) (-23.234239, 45.824651) (-23.205695, 45.824033) (-23.163932, 45.8181) (-23.124065, 45.808763) (-23.086179, 45.795718) (-23.050202, 45.779037) (-23.016466, 45.7582) (-22.984465, 45.733859) (-22.954772, 45.705874) (-22.927834, 45.675074) (-22.90415, 45.641959) (-22.884032, 45.606848) (-22.867852, 45.569408) (-22.854932, 45.530052) (-22.846333, 45.488365) (-22.840607, 45.444742) (-22.839967, 45.414914) (-22.839641, 45.399704) knots 0 0 0 0 0.06580765 0.12939427 0.19089406 0.25128107 0.31081496 0.37037099 0.43076826 0.49288125 0.55510395 0.61606705 0.67725603 0.73825981 0.80076213 0.86477758 0.93104529 1 1 1 1
  spline S8 degree 3 poles (-22.839641, 45.399704) (-22.839888, 45.38911) (-22.840379, 45.368066) (-22.842874, 45.336812) (-22.847679, 45.30622) (-22.85413, 45.276286) (-22.862503, 45.247066) (-22.872639, 45.218476) (-22.885043, 45.190695) (-22.898649, 45.16346) (-22.913969, 45.137387) (-22.930972, 45.113003) (-22.948937, 45.089943) (-22.968266, 45.068454) (-22.989141, 45.048678) (-23.011308, 45.030498) (-23.03459, 45.013604) (-23.059348, 44.998685) (-23.085029, 44.984956) (-23.112005, 44.973693) (-23.139662, 44.963623) (-23.168398, 44.955597) (-23.198147, 44.949307) (-23.228959, 44.945036) (-23.260671, 44.941925) (-23.282168, 44.94173) (-23.293026, 44.941631) knots 0 0 0 0 0.04401447 0.08743412 0.1301184 0.17255369 0.21455476 0.25629809 0.29843823 0.340849 0.38271519 0.42392405 0.46424624 0.50407367 0.54386191 0.58356672 0.62309432 0.66322906 0.70355126 0.74393789 0.78454125 0.82575011 0.86775736 0.91074516 0.95491445 1 1 1 1
  spline S9 degree 3 poles (-23.293026, 44.941631) (-23.30598, 44.941888) (-23.331464, 44.942393) (-23.3688, 44.947674) (-23.404722, 44.955238) (-23.438942, 44.966617) (-23.471766, 44.980875) (-23.502751, 44.998895) (-23.532691, 45.019316) (-23.560367, 45.043415) (-23.586053, 45.069755) (-23.609047, 45.098339) (-23.629525, 45.128696) (-23.64716, 45.160972) (-23.662202, 45.195084) (-23.674019, 45.231158) (-23.683557, 45.269006) (-23.687592, 45.295063) (-23.689641, 45.308298) knots 0 0 0 0 0.06542114 0.12870837 0.19023614 0.2507244 0.31063718 0.37076641 0.43161474 0.49352297 0.55588346 0.61734237 0.67866804 0.74071136 0.80298536 0.86680258 0.93234717 1 1 1 1
  line L36 (-23.689641, 45.308298) -> (-23.572974, 45.308298)
  spline S10 degree 3 poles (-23.572974, 45.308298) (-23.570104, 45.295901) (-23.564586, 45.272073) (-23.552475, 45.238596) (-23.537668, 45.208763) (-23.520061, 45.18218) (-23.499057, 45.159) (-23.475088, 45.138342) (-23.448216, 45.119706) (-23.418356, 45.104171) (-23.386854, 45.090923) (-23.353883, 45.082101) (-23.320342, 45.075898) (-23.297656, 45.075277) (-23.286256, 45.074965) knots 0 0 0 0 0.09468725 0.18199416 0.26437695 0.34217986 0.41861761 0.49650908 0.57736909 0.66151059 0.74673255 0.83125798 0.91520562 1 1 1 1
  spline S11 degree 3 poles (-23.286256, 45.074965) (-23.275128, 45.07527) (-23.253218, 45.07587) (-23.220974, 45.08049) (-23.189843, 45.087606) (-23.160134, 45.098255) (-23.131325, 45.111197) (-23.104146, 45.127805) (-23.077811, 45.146919) (-23.053138, 45.168817) (-23.03054, 45.192949) (-23.010574, 45.218755) (-22.993942, 45.246284) (-22.979927, 45.27506) (-22.969284, 45.305397) (-22.961692, 45.337155) (-22.957233, 45.370411) (-22.95662, 45.393094) (-22.956308, 45.404652) knots 0 0 0 0 0.0642073 0.12642469 0.18768028 0.24821642 0.30830506 0.36966099 0.43169855 0.49594689 0.55975802 0.62229541 0.68391064 0.74509241 0.80674023 0.86908662 0.93329 1 1 1 1
  spline S12 degree 3 poles (-22.956308, 45.404652) (-22.956552, 45.41508) (-22.957031, 45.435492) (-22.960942, 45.465355) (-22.967746, 45.49361) (-22.977189, 45.520396) (-22.989178, 45.545736) (-23.00383, 45.569657) (-23.021418, 45.591844) (-23.04151, 45.612307) (-23.06352, 45.631192) (-23.087827, 45.647291) (-23.113924, 45.660835) (-23.141495, 45.672523) (-23.171196, 45.680918) (-23.202439, 45.68722) (-23.235562, 45.690866) (-23.258209, 45.691371) (-23.269849, 45.691631) knots 0 0 0 0 0.06535138 0.12791603 0.18836021 0.24721608 0.30563013 0.36376984 0.42266091 0.48268729 0.54330022 0.60411796 0.66496489 0.72741349 0.79146763 0.85805544 0.92703681 1 1 1 1
  spline S13 degree 3 poles (-23.269849, 45.691631) (-23.279926, 45.691416) (-23.300731, 45.690971) (-23.332645, 45.687692) (-23.366182, 45.682403) (-23.401213, 45.675128) (-23.437844, 45.665608) (-23.475996, 45.6542) (-23.515751, 45.64056) (-23.542538, 45.63026) (-23.556308, 45.624965) knots 0 0 0 0 0.10220304 0.21102334 0.32509966 0.4465021 0.57378772 0.70890071 0.85035787 1 1 1 1
  line L37 (-20.109641, 44.974965) -> (-19.492974, 46.274965)
  line L38 (-19.492974, 46.274965) -> (-19.476308, 46.274965)
  line L39 (-19.476308, 46.274965) -> (-18.876308, 44.974965)
  line L40 (-18.876308, 44.974965) -> (-19.003131, 44.974965)
  line L41 (-19.003131, 44.974965) -> (-19.195318, 45.391631)
  line L42 (-19.195318, 45.391631) -> (-19.784641, 45.391631)
  line L43 (-19.784641, 45.391631) -> (-19.982297, 44.974965)
  line L44 (-19.982297, 44.974965) -> (-20.109641, 44.974965)
  spline S14 degree 3 poles (-18.599641, 45.632517) (-18.599063, 45.6559) (-18.597927, 45.701906) (-18.588271, 45.769422) (-18.572739, 45.834107) (-18.550677, 45.895839) (-18.522706, 45.954945) (-18.488154, 46.010972) (-18.44742, 46.064278) (-18.400825, 46.114055) (-18.349729, 46.159569) (-18.29501, 46.199612) (-18.236777, 46.232935) (-18.17567, 46.260791) (-18.111233, 46.282202) (-18.043602, 46.29719) (-17.972905, 46.306519) (-17.92467, 46.307699) (-17.900162, 46.308298) knots 0 0 0 0 0.06455785 0.12701353 0.18795481 0.24801391 0.30774768 0.36823451 0.42946984 0.49274344 0.55625777 0.61821679 0.67965548 0.74124555 0.80341526 0.86681546 0.93232831 1 1 1 1
  spline S15 degree 3 poles (-17.900162, 46.308298) (-17.885225, 46.308119) (-17.855659, 46.307765) (-17.811922, 46.304308) (-17.769341, 46.298546) (-17.727885, 46.290703) (-17.687354, 46.280969) (-17.648057, 46.268288) (-17.609763, 46.253789) (-17.572714, 46.23709) (-17.537088, 46.218345) (-17.502896, 46.197762) (-17.470409, 46.175366) (-17.439399, 46.151349) (-17.410384, 46.125201) (-17.382541, 46.097641) (-17.356816, 46.067877) (-17.340936, 46.046927) (-17.332974, 46.036423) knots 0 0 0 0 0.06854754 0.13568295 0.20121499 0.26568223 0.32926683 0.39239543 0.45506976 0.51712685 0.57879004 0.63973986 0.7001915 0.75980624 0.81962832 0.87935479 0.93951161 1 1 1 1
  line L45 (-17.332974, 46.036423) -> (-17.435058, 45.958298)
  spline S16 degree 3 poles (-17.435058, 45.958298) (-17.44234, 45.966977) (-17.456806, 45.984217) (-17.480079, 46.008427) (-17.504334, 46.031108) (-17.529561, 46.05237) (-17.556215, 46.071467) (-17.583649, 46.089397) (-17.612322, 46.105467) (-17.651973, 46.124954) (-17.703842, 46.145288) (-17.769137, 46.162338) (-17.837299, 46.173191) (-17.883801, 46.174367) (-17.907453, 46.174965) knots 0 0 0 0 0.06316326 0.12547494 0.18712122 0.24829435 0.30929486 0.36985007 0.43097338 0.49245599 0.61614797 0.7408437 0.86818265 1 1 1 1
  spline S17 degree 3 poles (-17.907453, 46.174965) (-17.920484, 46.174815) (-17.946425, 46.174516) (-17.984923, 46.170575) (-18.022702, 46.165037) (-18.059738, 46.156819) (-18.095983, 46.146429) (-18.131675, 46.134014) (-18.166296, 46.118654) (-18.200325, 46.101676) (-18.232929, 46.0825) (-18.263778, 46.061584) (-18.29276, 46.039161) (-18.319897, 46.015148) (-18.345219, 45.989652) (-18.36854, 45.962403) (-18.38978, 45.933486) (-18.40936, 45.903284) (-18.426897, 45.871884) (-18.441579, 45.839171) (-18.454581, 45.805704) (-18.464869, 45.771105) (-18.473013, 45.735617) (-18.478632, 45.699146) (-18.482527, 45.661768) (-18.482824, 45.636433) (-18.482974, 45.623663) knots 0 0 0 0 0.04395491 0.08750187 0.13046263 0.17275202 0.21540307 0.25764983 0.30015275 0.34312149 0.38592516 0.42768573 0.46881795 0.5094918 0.54988303 0.58998002 0.63040523 0.67086863 0.71138394 0.75162726 0.79177558 0.83245892 0.87331905 0.91454296 0.95692356 1 1 1 1
  spline S18 degree 3 poles (-18.482974, 45.623663) (-18.482506, 45.604448) (-18.481585, 45.566723) (-18.473396, 45.511465) (-18.460951, 45.458529) (-18.4423, 45.408245) (-18.419301, 45.359994) (-18.39024, 45.314591) (-18.356583, 45.27135) (-18.317852, 45.231294) (-18.275359, 45.194703) (-18.229767, 45.162482) (-18.18119, 45.135622) (-18.130164, 45.113271) (-18.076297, 45.09609) (-18.019686, 45.083995) (-17.960454, 45.076105) (-17.919979, 45.075349) (-17.899381, 45.074965) knots 0 0 0 0 0.06432322 0.1262901 0.18672647 0.24614643 0.30557564 0.36542939 0.42632631 0.48883991 0.55172497 0.6139186 0.67548377 0.7373339 0.80022904 0.8645023 0.93104074 1 1 1 1
  spline S19 degree 3 poles (-17.899381, 45.074965) (-17.876685, 45.075592) (-17.832015, 45.076827) (-17.766507, 45.087286) (-17.703797, 45.104244) (-17.643881, 45.127978) (-17.586928, 45.158831) (-17.532849, 45.196233) (-17.481599, 45.24054) (-17.450781, 45.274371) (-17.435058, 45.291631) knots 0 0 0 0 0.12851519 0.25294864 0.37475473 0.49593975 0.61718064 0.74090947 0.86781115 1 1 1 1
  line L46 (-17.435058, 45.291631) -> (-17.332974, 45.214288)
  spline S20 degree 3 poles (-17.332974, 45.214288) (-17.34119, 45.203688) (-17.357581, 45.182538) (-17.384122, 45.152723) (-17.412083, 45.124679) (-17.441669, 45.098631) (-17.472541, 45.07406) (-17.505254, 45.051662) (-17.539377, 45.031125) (-17.574794, 45.012321) (-17.611468, 44.995638) (-17.649356, 44.981355) (-17.688293, 44.969051) (-17.728281, 44.958929) (-17.769404, 44.951028) (-17.811513, 44.945747) (-17.854699, 44.942128) (-17.883835, 44.941799) (-17.898599, 44.941631) knots 0 0 0 0 0.06167424 0.12305306 0.183475 0.2437265 0.30427892 0.36486292 0.4259462 0.48739123 0.54922038 0.61114359 0.67352853 0.73696146 0.80078528 0.8660126 0.93210075 1 1 1 1
  spline S21 degree 3 poles (-17.898599, 44.941631) (-17.912581, 44.941729) (-17.940229, 44.941921) (-17.981048, 44.945038) (-18.020787, 44.949291) (-18.059332, 44.955694) (-18.096893, 44.963251) (-18.13313, 44.97338) (-18.168399, 44.984727) (-18.202559, 44.998063) (-18.235638, 45.013112) (-18.26753, 45.03012) (-18.298221, 45.048945) (-18.328011, 45.069171) (-18.356462, 45.091449) (-18.383819, 45.115468) (-18.410236, 45.141147) (-18.42658, 45.159665) (-18.434797, 45.168975) knots 0 0 0 0 0.0696628 0.13774956 0.20391674 0.26877986 0.33241371 0.39475354 0.45618003 0.51699565 0.57739594 0.63719834 0.69699918 0.75675619 0.81655391 0.876948 0.93813179 1 1 1 1
  spline S22 degree 3 poles (-18.434797, 45.168975) (-18.447959, 45.185148) (-18.474124, 45.217297) (-18.507599, 45.269403) (-18.536254, 45.323806) (-18.559422, 45.38079) (-18.577534, 45.440229) (-18.590081, 45.502152) (-18.598235, 45.566501) (-18.599167, 45.610269) (-18.599641, 45.632517) knots 0 0 0 0 0.12432851 0.24715602 0.36877975 0.49073386 0.61361377 0.73895758 0.86731058 1 1 1 1
  line L47 (-15.526977, 46.224965) -> (-15.739813, 46.224965)
  line L48 (-15.927345, 45.124965) -> (-15.526977, 46.224965)
  line L49 (-15.427345, 45.124965) -> (-15.927345, 45.124965)
  line L50 (-15.026977, 46.224965) -> (-15.427345, 45.124965)
  line L51 (-14.814142, 46.224965) -> (-15.026977, 46.224965)
  line L52 (-15.214509, 45.124965) -> (-14.814142, 46.224965)
  line L53 (-15.014509, 45.124965) -> (-15.214509, 45.124965)
  line L54 (-15.087303, 44.924965) -> (-15.014509, 45.124965)
  line L55 (-16.212974, 44.924965) -> (-15.087303, 44.924965)
  line L56 (-15.739813, 46.224965) -> (-16.212974, 44.924965)
  line L57 (-20.902974, 44.974965) -> (-20.919641, 44.974965)
  line L58 (-20.919641, 44.974965) -> (-21.469641, 46.274965)
  line L59 (-21.469641, 46.274965) -> (-21.344641, 46.274965)
  line L60 (-21.344641, 46.274965) -> (-20.911308, 45.250486)
  line L61 (-20.911308, 45.250486) -> (-20.477974, 46.274965)
  line L62 (-20.477974, 46.274965) -> (-20.352974, 46.274965)
  line L63 (-20.352974, 46.274965) -> (-20.902974, 44.974965)
  spline S23 degree 3 poles (-21.712974, 45.624444) (-21.713216, 45.604564) (-21.713688, 45.565828) (-21.716131, 45.509173) (-21.720945, 45.455688) (-21.726965, 45.405244) (-21.735304, 45.358052) (-21.745558, 45.313947) (-21.756942, 45.272739) (-21.770995, 45.234766) (-21.786376, 45.199498) (-21.803111, 45.166564) (-21.82104, 45.135674) (-21.840573, 45.107074) (-21.861393, 45.080562) (-21.883945, 45.056606) (-21.907594, 45.034628) (-21.932633, 45.015072) (-21.958786, 44.997955) (-21.985513, 44.982647) (-22.01329, 44.970303) (-22.041486, 44.959704) (-22.070505, 44.951607) (-22.100311, 44.946008) (-22.130752, 44.942082) (-22.15133, 44.941782) (-22.161672, 44.941631) knots 0 0 0 0 0.06506329 0.12677317 0.18551576 0.24076468 0.2929798 0.34225037 0.38891929 0.43277566 0.47462843 0.51477469 0.55360589 0.59142641 0.62802812 0.66380363 0.69898434 0.73359149 0.76762847 0.80120835 0.83426384 0.86698069 0.89971974 0.93270191 0.96617588 1 1 1 1